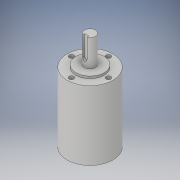
# Autodesk Inventor part: 19_1 Chinesium
Saved by Autodesk Inventor 2019.4 (Build 234330000, 330)
## iProperties
Created: 2020-02-13
Part Number: 19_1 Chinesium
Material: Generic
Document SubType Name: Modeling
Designer: admin
Appearance: Default
Surface Area: 126.064 cm^2
Volume: 90.3535 cm^3
Author: admin
Autodesk Inventor part; units mm, degrees
ref_plane "YZ Plane" through (0, 0, 0) normal (1, 0, 0) x (0, 1, 0)
ref_plane "XZ Plane" through (0, 0, 0) normal (0, 1, 0) x (-1, 0, 0)
ref_plane "XY Plane" through (0, 0, 0) normal (0, 0, 1) x (1, 0, 0)
sketch "Sketch1" plane through (0, 0, 0) normal (0, 1, 0) x (-1, 0, 0)
  circle A0 centre (0, 0) radius 21
  dimension "d0" = 42
  constraints: 1 centre point, 1 coincident
  measures "d0" diameter of A0
extrude "Extrusion1" add sketch "Sketch1" along normal blind 63.5
sketch "Sketch2" plane through (0, 63.5, 0) normal (0, 1, 0) x (1, 0, 0)
  circle A0 centre (0, 0) radius 13
  dimension "d3" = 26
  constraints: 1 centre point, 1 coincident
  measures "d3" diameter of A0
extrude "Extrusion2" add sketch "Sketch2" along normal blind 2
sketch "Sketch3" plane through (0, 65.5, 0) normal (0, 1, 0) x (1, 0, 0)
  circle A0 centre (0, 0) radius 5
  dimension "d6" = 10
  constraints: 1 centre point, 1 coincident
  measures "d6" diameter of A0
extrude "Extrusion3" add sketch "Sketch3" along normal blind 25
sketch "Sketch4" plane through (0, 90.5, 0) normal (0, 1, 0) x (1, 0, 0)
  line L0 (-2.1218, -6.8094) -> (-2.1218, -2.8094)
  line L1 (-2.1218, -2.8094) -> (1.8782, -2.8094)
  line L2 (1.8782, -2.8094) -> (1.8782, -6.8094)
  line L3 (1.8782, -6.8094) -> (-2.1218, -6.8094)
  point P0 (0, 0)
  dimension "d9" = 4
  dimension "d10" = 4
  constraints: 8 end point, 3 perpendicular, 1 vertical
  measures "d9" distance of L0.end L1.end
  measures "d10" distance of L0.start L0.end
extrude "Extrusion4" cut sketch "Sketch4" against normal blind 20
fillet "Fillet1" radius 2 2 edges at (-2.1218, 70.5, 3.6684) (1.8782, 70.5, 3.7216)
sketch "Sketch5" plane through (0, 63.5, 0) normal (0, 1, 0) x (1, 0, 0)
  circle A0 centre (0, 0) radius 17 construction
  circle A1 centre (0, -17) radius 2.2
  circle A2 centre (17, 0) radius 2.2
  circle A3 centre (0, 17) radius 2.2
  circle A4 centre (-17, 0) radius 2.2
  dimension "d14" = 34
  dimension "d15" = 4.4
  dimension "d18" = 360
  constraints: 4 centre point, 1 coincident, 1 vertical alignment, 11 other
  measures "d15" diameter of A1
extrude "Extrusion5" cut sketch "Sketch5" against normal blind 8
body "Solid1"
